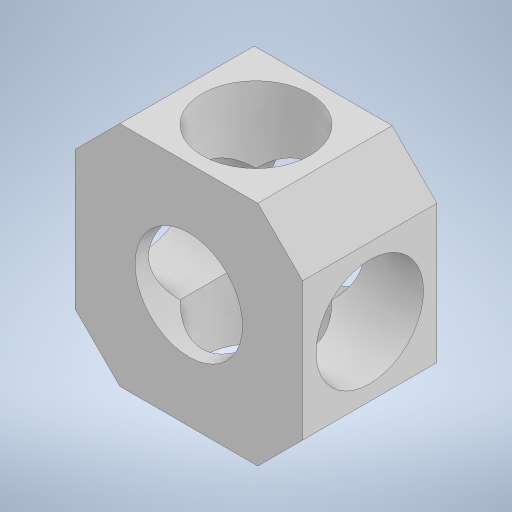
# Autodesk Inventor part: nut
Saved by Autodesk Inventor 2024 (Build 280153000, 153)
## iProperties
Created: 2023-10-30
Part Number: nut
Material: Generic
Document SubType Name: Modeling
Designer: Admin
Density: 1 g/cm^3
Appearance: Default
Author: Admin
Autodesk Inventor part; units mm, degrees
ref_plane "YZ Plane" through (0, 0, 0) normal (1, 0, 0) x (0, 1, 0)
ref_plane "XZ Plane" through (0, 0, 0) normal (0, 1, 0) x (-1, 0, 0)
ref_plane "XY Plane" through (0, 0, 0) normal (0, 0, 1) x (1, 0, 0)
sketch "Sketch1" plane through (0, 0, 0) normal (0, 0, 1) x (1, 0, 0)
  line L0 (-12.7, 12.7) -> (12.7, 12.7)
  line L1 (12.7, 12.7) -> (12.7, -12.7)
  line L2 (12.7, -12.7) -> (-12.7, -12.7)
  line L3 (-12.7, -12.7) -> (-12.7, 12.7)
  line L4 (-12.7, 12.7) -> (12.7, -12.7) construction
  line L5 (12.7, 12.7) -> (-12.7, -12.7) construction
  line L6 (7.7, -12.7) -> (12.7, -7.7)
  line L7 (0, -18.7345) -> (0, 15.4172) construction
  line L8 (-17.0055, 0) -> (21.2173, 0) construction
  line L9 (-7.7, -12.7) -> (-12.7, -7.7)
  line L10 (7.7, 12.7) -> (12.7, 7.7)
  line L11 (-7.7, 12.7) -> (-12.7, 7.7)
  circle A0 centre (0, 0) radius 6
  dimension "d0" = 25.4
  dimension "d1" = 25.4
  dimension "d2" = 5
  dimension "d3" = 5
  dimension "d4" = 12
  dimension "d14" = 12.7
  dimension "d15" = 28.85
  dimension "d16" = 8.5173
  dimension "d17" = 0
  dimension "d18" = 0
  dimension "d19" = 5
  dimension "d20" = 0
  dimension "d21" = 3.5234
  dimension "d22" = 27.6723
  dimension "d23" = 20.4
  dimension "d24" = 10.8894
  dimension "d25" = 20.4
  dimension "d26" = 28.85
  dimension "d27" = 25.4
  dimension "d28" = 17.9605
  dimension "d29" = 25.4
  dimension "d30" = 28.85
  dimension "d31" = 29.7055
  constraints: 24 end point, 6 symmetric about line, 2 horizontal, 2 midpoint, 2 parallel, 2 point on line, 1 centre point, 1 coincident, 1 perpendicular, 1 vertical
  measures "d0" distance of L1.end L2.end
  measures "d1" distance of L0.end L1.end
  measures "d2" distance of L1.end L6.end
  measures "d3" distance of L1.end L6.start
  measures "d4" diameter of A0
  measures "d14" distance between parallel lines of L7 L1
  measures "d15" distance between parallel lines of L10 L9
  measures "d16" distance from line of L8.end L1
  measures "d17" distance from line of point (12.7, 7.7) L1
  measures "d18" distance from line of point (12.7, 7.7) L10
  measures "d19" distance from line of point (7.7, 12.7) L1
  measures "d20" distance from line of point (7.7, 12.7) L10
  measures "d21" distance from line of L7.end L10
  measures "d22" distance from line of L7.start L10
  measures "d23" distance from line of point (-7.7, 12.7) L1
  measures "d24" distance from line of point (-7.7, 12.7) L10
  measures "d25" distance from line of point (-7.7, -12.7) L1
  measures "d26" distance from line of point (-7.7, -12.7) L10
  measures "d27" distance from line of point (-12.7, 7.7) L1
  measures "d28" distance from line of point (-12.7, 7.7) L10
  measures "d29" distance from line of point (-12.7, -7.7) L1
  measures "d30" distance from line of point (-12.7, -7.7) L10
  measures "d31" distance from line of L8.start L1
extrude "Extrusion1" add sketch "Sketch1" against normal blind 15 contours L0 L10 L1 L6 L2 L9 L3 L11
sketch "Sketch2" plane through (-7.7, 12.7, 0) normal (0, 1, 0) x (1, 0, 0)
  line L0 (15.4, 0) -> (0, 0) projected
  circle A0 centre (7.7, 7.5) radius 6
  point P0 (7.7, 0)
  point P1 (7.7, 0)
  dimension "d7" = 7.5
  dimension "d8" = 12
  dimension "d32" = 7.5
  constraints: 1 centre point, 1 coincident, 1 midpoint
  measures "d7" distance of point (7.7, 0) point (7.7, 7.5)
  measures "d8" diameter of A0
  measures "d32" distance from line of point (7.7, 7.5) L0
extrude "Extrusion2" cut sketch "Sketch2" against normal through all
pattern_circular "Circular Pattern1" count 4 over 360 about axis through (0, 0, -10) along (0, 0, 1) of "Extrusion2"
body "Solid1"
